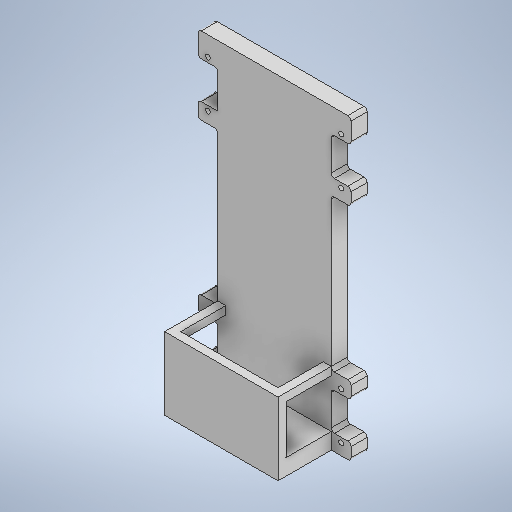
# Autodesk Inventor part: Internal frame
Saved by Autodesk Inventor 2025.1 (Build 291241020, 241B)
## iProperties
Created: 2026-04-23
Part Number: Internal frame
Material: Generic
Document SubType Name: Modeling
Designer: Owner
Density: 1 g/cm^3
Appearance: Default
Author: Owner
Autodesk Inventor part; units mm, degrees
ref_plane "YZ Plane" through (0, 0, 0) normal (1, 0, 0) x (0, 1, 0)
ref_plane "XZ Plane" through (0, 0, 0) normal (0, 1, 0) x (-1, 0, 0)
ref_plane "XY Plane" through (0, 0, 0) normal (0, 0, 1) x (1, 0, 0)
sketch "Sketch1" plane through (0, 0, 0) normal (0, 0, 1) x (1, 0, 0)
  line L0 (0, 0) -> (95, 0)
  line L1 (95, 0) -> (95, 185)
  line L2 (95, 185) -> (0, 185)
  line L3 (0, 185) -> (0, 0)
  line L4 (0, 185) -> (95, 185)
  line L5 (95, 185) -> (95, 170)
  line L6 (95, 170) -> (0, 170)
  line L7 (0, 170) -> (0, 185)
  line L8 (0, 0) -> (95, 0)
  line L9 (95, 0) -> (95, 10)
  line L10 (95, 10) -> (0, 10)
  line L11 (0, 10) -> (0, 0)
  line L12 (0, 170) -> (12.3, 170)
  line L13 (12.3, 170) -> (12.3, 147)
  line L14 (12.3, 147) -> (0, 147)
  line L15 (0, 147) -> (0, 170)
  line L16 (95, 170) -> (82.7, 170)
  line L17 (82.7, 170) -> (82.7, 147)
  line L18 (82.7, 147) -> (95, 147)
  line L19 (95, 147) -> (95, 170)
  line L20 (0, 10) -> (12.3, 10)
  line L21 (12.3, 10) -> (12.3, 33)
  line L22 (12.3, 33) -> (0, 33)
  line L23 (0, 33) -> (0, 10)
  line L24 (95, 10) -> (82.7, 10)
  line L25 (82.7, 10) -> (82.7, 33)
  line L26 (82.7, 33) -> (95, 33)
  line L27 (95, 33) -> (95, 10)
  circle A0 centre (6.15, 173) radius 1.5
  circle A1 centre (88.85, 173) radius 1.5
  circle A2 centre (6.15, 7) radius 1.5
  circle A3 centre (88.85, 7) radius 1.5
  line L28 (12.3, 10) -> (12.3, 0)
  line L29 (82.7, 10) -> (82.7, 0)
  line L30 (12.3, 170) -> (82.7, 170)
  line L31 (82.7, 170) -> (82.7, 10)
  line L32 (82.7, 10) -> (12.3, 10)
  line L33 (12.3, 10) -> (12.3, 170)
  line L34 (82.7, 137) -> (95, 137)
  line L35 (12.3, 137) -> (0, 137)
  line L36 (0, 43) -> (12.3, 43)
  line L37 (82.7, 43) -> (95, 43)
  circle A4 centre (6.15, 36) radius 1.5
  circle A5 centre (88.85, 36) radius 1.5
  circle A6 centre (6.15, 144) radius 1.5
  circle A7 centre (88.85, 144) radius 1.5
  point P0 (88.85, 10)
  point P1 (0, 170)
  point P2 (0, 147)
  point P3 (0, 33)
  point P4 (0, 10)
  dimension "d0" = 185
  dimension "d1" = 95
  dimension "d2" = 15
  dimension "d3" = 10
  dimension "d4" = 23
  dimension "d5" = 12.3
  dimension "d6" = 12.3
  dimension "d7" = 23
  dimension "d8" = 23
  dimension "d9" = 12.3
  dimension "d10" = 23
  dimension "d11" = 12.3
  dimension "d12" = 3
  dimension "d13" = 6.15
  dimension "d14" = 3
  dimension "d15" = 3
  dimension "d16" = 6.15
  dimension "d17" = 3
  dimension "d18" = 3
  dimension "d19" = 6.15
  dimension "d20" = 3
  dimension "d21" = 3
  dimension "d22" = 3
  dimension "d23" = 6.15
  dimension "d24" = 10
  dimension "d25" = 10
  dimension "d26" = 3
  dimension "d27" = 3
  dimension "d28" = 6.15
  dimension "d29" = 3
  dimension "d30" = 3
  dimension "d31" = 6.15
  dimension "d32" = 3
  dimension "d33" = 3
  dimension "d34" = 6.15
  dimension "d35" = 3
  dimension "d36" = 6.15
  dimension "d37" = 3
  constraints: 76 end point, 16 parallel, 16 point on line, 12 perpendicular, 8 centre point, 8 horizontal, 1 midpoint
  measures "d0" distance between parallel lines of L0 L2
  measures "d1" distance between parallel lines of L1 L3
  measures "d2" distance between parallel lines of L6 L2
  measures "d3" distance between parallel lines of L0 L10
  measures "d4" distance between parallel lines of L14 L6
  measures "d5" distance from line of L6.end L13
  measures "d6" distance from line of L5.end L17
  measures "d7" distance from line of L5.end L18
  measures "d8" distance from line of L10.end L22
  measures "d9" distance from line of L10.end L21
  measures "d10" distance from line of point (88.85, 10) L26
  measures "d11" distance between parallel lines of L1 L25
  measures "d12" vertical distance of L6.end A0.centre
  measures "d13" horizontal distance of L6.end A0.centre
  measures "d14" diameter of A0
  measures "d15" vertical distance of L5.end A1.centre
  measures "d16" horizontal distance of L5.end A1.centre
  measures "d17" diameter of A1
  measures "d18" vertical distance of L10.end A2.centre
  measures "d19" horizontal distance of L10.end A2.centre
  measures "d20" diameter of A2
  measures "d21" diameter of A3
  measures "d22" vertical distance of L9.end A3.centre
  measures "d23" horizontal distance of L9.end A3.centre
  measures "d24" distance between parallel lines of L34 L18
  measures "d25" distance between parallel lines of L26 L37
  measures "d26" diameter of A4
  measures "d27" vertical distance of L22.end A4.centre
  measures "d28" horizontal distance of L22.end A4.centre
  measures "d29" diameter of A5
  measures "d30" vertical distance of L26.end A5.centre
  measures "d31" horizontal distance of L26.end A5.centre
  measures "d32" diameter of A6
  measures "d33" vertical distance of L14.end A6.centre
  measures "d34" horizontal distance of L14.end A6.centre
  measures "d35" diameter of A7
  measures "d36" horizontal distance of L18.end A7.centre
  measures "d37" vertical distance of L18.end A7.centre
extrude "Extrusion1" add sketch "Sketch1" along normal blind 10 contours L3 L10 L28 L0 | L28 L10 L29 L0 | L29 L10 L1 L0 | L21 L33 L13 L6 L17 L31 L25 L10 | L3 L36 L33 L22 | L31 L37 L1 L26 | L3 L14 L33 L35 | L31 L18 L1 L34 | L3 L2 L1 L6
sketch "Sketch2" plane through (0, 0, 10) normal (0, 0, 1) x (1, 0, 0)
  line L0 (12.3, 10) -> (82.7, 10)
  line L1 (82.7, 10) -> (82.7, 0)
  line L2 (82.7, 0) -> (12.3, 0)
  line L3 (12.3, 0) -> (12.3, 10)
  line L4 (0, 10) -> (0, 0) projected
  dimension "d45" = 5
  dimension "d40" = 10
  dimension "d41" = 70.4
  dimension "d42" = 12.3
  constraints: 8 end point, 2 parallel, 1 horizontal, 1 perpendicular
  measures "d40" distance between parallel lines of L2 L0
  measures "d41" distance between parallel lines of L3 L1
  measures "d42" distance between parallel lines of L4 L3
extrude "Extrusion2" add sketch "Sketch2" along normal blind 33
sketch "Sketch3" plane through (12.3, 10, 10) normal (0, 1, 0) x (1, 0, 0)
  line L0 (0, -33) -> (70.4, -33) projected
  line L1 (0, -33) -> (70.4, -33)
  line L2 (70.4, -33) -> (70.4, -28)
  line L3 (70.4, -28) -> (0, -28)
  line L4 (0, -28) -> (0, -33)
  point P0 (-12.3, 10)
  dimension "d45" = 5
  constraints: 8 end point, 2 parallel, 1 horizontal, 1 perpendicular
  measures "d45" distance between parallel lines of L0 L3
extrude "Extrusion3" add sketch "Sketch3" along normal blind 35
fillet "Fillet1" radius 2 27 edges at (0, 185, 5) (0, 170, 5) (0, 147, 5) (0, 137, 5) (0, 43, 5) (0, 33, 5) (0, 10, 5) (0, 0, 5) (12.3, 43, 5) (12.3, 10, 5) (12.3, 33, 5) (12.3, 170, 5) (12.3, 137, 5) (95, 0, 5) (95, 10, 5) (82.7, 10, 5) (95, 33, 5) (95, 43, 5) (82.7, 43, 5) (95, 137, 5) (95, 147, 5) (82.7, 147, 5) (95, 170, 5) (95, 185, 5) (82.7, 137, 5) (82.7, 170, 5) (82.7, 33, 5)
sketch "Sketch4" plane through (82.7, 10, 38) normal (0, 0, -1) x (-1, 0, 0)
  line L0 (0, 35) -> (70.4, 35) projected
  line L1 (70.4, 0) -> (70.4, 35) projected
  line L2 (65.4, 35) -> (70.4, 35)
  line L3 (70.4, 35) -> (70.4, 30)
  line L4 (70.4, 30) -> (65.4, 30)
  line L5 (65.4, 30) -> (65.4, 35)
  line L6 (5, 35) -> (0, 35)
  line L7 (0, 35) -> (0, 30)
  line L8 (0, 30) -> (5, 30)
  line L9 (5, 30) -> (5, 35)
  point P0 (82.7, -10)
  dimension "d49" = 5
  dimension "d50" = 5
  dimension "d51" = 5
  dimension "d52" = 5
  constraints: 16 end point, 4 parallel, 3 point on line, 2 horizontal, 2 perpendicular
  measures "d49" distance between parallel lines of L0 L4
  measures "d50" distance between parallel lines of L1 L5
  measures "d51" distance between parallel lines of L0 L8
  measures "d52" distance between parallel lines of L7 L9
extrude "Extrusion4" add sketch "Sketch4" along normal blind 29
body "Solid1"
